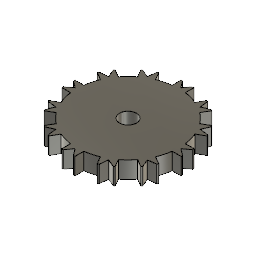
turn wheel v2 (Autodesk Fusion 360 design; units mm, degrees)
Autodesk Fusion 360 part; units mm, degrees
sketch "turn wheel" plane through (0, 0, 0) normal (0, 0, 1) x (1, 0, 0)
  circle A0 centre (0, 0) radius 30
  line L0 (-3.8635, 29.7502) -> (-3.8635, 35)
  line L1 (-3.8635, 35) -> (-3, 35)
  line L2 (-3, 35) -> (0, 31)
  line L3 (0, 35) -> (0, 30) construction
  line L4 (3.8635, 29.7502) -> (3.8635, 35)
  line L5 (3.8635, 35) -> (3, 35)
  line L6 (3, 35) -> (0, 31)
  line L7 (-18.2209, 23.8327) -> (-20.8458, 28.3792)
  line L8 (-20.0981, 28.8109) -> (-15.5, 26.8468)
  line L9 (-20.8458, 28.3792) -> (-20.0981, 28.8109)
  line L10 (-14.9019, 31.8109) -> (-15.5, 26.8468)
  line L11 (-14.1542, 32.2426) -> (-14.9019, 31.8109)
  line L12 (-11.5292, 27.6961) -> (-14.1542, 32.2426)
  line L13 (-27.6961, 11.5292) -> (-32.2426, 14.1542)
  line L14 (-31.8109, 14.9019) -> (-26.8468, 15.5)
  line L15 (-32.2426, 14.1542) -> (-31.8109, 14.9019)
  line L16 (-28.8109, 20.0981) -> (-26.8468, 15.5)
  line L17 (-28.3792, 20.8458) -> (-28.8109, 20.0981)
  line L18 (-23.8327, 18.2209) -> (-28.3792, 20.8458)
  line L19 (-29.7502, -3.8635) -> (-35, -3.8635)
  line L20 (-35, -3) -> (-31, 0)
  line L21 (-35, -3.8635) -> (-35, -3)
  line L22 (-35, 3) -> (-31, 0)
  line L23 (-35, 3.8635) -> (-35, 3)
  line L24 (-29.7502, 3.8635) -> (-35, 3.8635)
  line L25 (-23.8327, -18.2209) -> (-28.3792, -20.8458)
  line L26 (-28.8109, -20.0981) -> (-26.8468, -15.5)
  line L27 (-28.3792, -20.8458) -> (-28.8109, -20.0981)
  line L28 (-31.8109, -14.9019) -> (-26.8468, -15.5)
  line L29 (-32.2426, -14.1542) -> (-31.8109, -14.9019)
  line L30 (-27.6961, -11.5292) -> (-32.2426, -14.1542)
  line L31 (-11.5292, -27.6961) -> (-14.1542, -32.2426)
  line L32 (-14.9019, -31.8109) -> (-15.5, -26.8468)
  line L33 (-14.1542, -32.2426) -> (-14.9019, -31.8109)
  line L34 (-20.0981, -28.8109) -> (-15.5, -26.8468)
  line L35 (-20.8458, -28.3792) -> (-20.0981, -28.8109)
  line L36 (-18.2209, -23.8327) -> (-20.8458, -28.3792)
  line L37 (3.8635, -29.7502) -> (3.8635, -35)
  line L38 (3, -35) -> (0, -31)
  line L39 (3.8635, -35) -> (3, -35)
  line L40 (-3, -35) -> (0, -31)
  line L41 (-3.8635, -35) -> (-3, -35)
  line L42 (-3.8635, -29.7502) -> (-3.8635, -35)
  line L43 (18.2209, -23.8327) -> (20.8458, -28.3792)
  line L44 (20.0981, -28.8109) -> (15.5, -26.8468)
  line L45 (20.8458, -28.3792) -> (20.0981, -28.8109)
  line L46 (14.9019, -31.8109) -> (15.5, -26.8468)
  line L47 (14.1542, -32.2426) -> (14.9019, -31.8109)
  line L48 (11.5292, -27.6961) -> (14.1542, -32.2426)
  line L49 (27.6961, -11.5292) -> (32.2426, -14.1542)
  line L50 (31.8109, -14.9019) -> (26.8468, -15.5)
  line L51 (32.2426, -14.1542) -> (31.8109, -14.9019)
  line L52 (28.8109, -20.0981) -> (26.8468, -15.5)
  line L53 (28.3792, -20.8458) -> (28.8109, -20.0981)
  line L54 (23.8327, -18.2209) -> (28.3792, -20.8458)
  line L55 (29.7502, 3.8635) -> (35, 3.8635)
  line L56 (35, 3) -> (31, 0)
  line L57 (35, 3.8635) -> (35, 3)
  line L58 (35, -3) -> (31, 0)
  line L59 (35, -3.8635) -> (35, -3)
  line L60 (29.7502, -3.8635) -> (35, -3.8635)
  line L61 (23.8327, 18.2209) -> (28.3792, 20.8458)
  line L62 (28.8109, 20.0981) -> (26.8468, 15.5)
  line L63 (28.3792, 20.8458) -> (28.8109, 20.0981)
  line L64 (31.8109, 14.9019) -> (26.8468, 15.5)
  line L65 (32.2426, 14.1542) -> (31.8109, 14.9019)
  line L66 (27.6961, 11.5292) -> (32.2426, 14.1542)
  line L67 (11.5292, 27.6961) -> (14.1542, 32.2426)
  line L68 (14.9019, 31.8109) -> (15.5, 26.8468)
  line L69 (14.1542, 32.2426) -> (14.9019, 31.8109)
  line L70 (20.0981, 28.8109) -> (15.5, 26.8468)
  line L71 (20.8458, 28.3792) -> (20.0981, 28.8109)
  line L72 (18.2209, 23.8327) -> (20.8458, 28.3792)
  dimension "d1" = 60
  dimension "d2" = 5.2498
  dimension "d3" = 0.8635
  dimension "d4" = 5
  dimension "d6" = 360
  constraint coincident A0.centre origin
  constraint coincident A0 L0.start
  constraint vertical L0
  constraint perpendicular L0 L1
  constraint coincident A0 L3.end
  constraint vertical L3
  constraint symmetric L0.start L3 L4.start
  constraint symmetric L0.end L3 L4.end
  constraint symmetric L1.end L3 L5.end
  constraint symmetric L2.end L3 L6.end
  constraint perpendicular L4 L5
  measures "d1" diameter of A0
  measures "d2" distance of L0.start L0.end
  measures "d3" distance of L0.end L1.end
  measures "d4" distance of L1.end L2.end
extrude "Extrude1" add sketch "turn wheel" along normal blind 10
sketch "hole punch" plane through (0, 0, 10) normal (0, 0, 1) x (-1, 0, 0)
  arc A0 (-23.8327, -18.2209) -> (-18.2209, -23.8327) centre (0, 0) ccw
  line L0 (-18.2209, -23.8327) -> (-20.8458, -28.3792)
  line L1 (-20.8458, -28.3792) -> (-20.0981, -28.8109)
  line L2 (-20.0981, -28.8109) -> (-15.5, -26.8468)
  line L3 (-15.5, -26.8468) -> (-14.9019, -31.8109)
  line L4 (-14.9019, -31.8109) -> (-14.1542, -32.2426)
  line L5 (-14.1542, -32.2426) -> (-11.5292, -27.6961)
  arc A1 (-11.5292, -27.6961) -> (-3.8635, -29.7502) centre (0, 0) ccw
  line L6 (-3.8635, -29.7502) -> (-3.8635, -35)
  line L7 (-3.8635, -35) -> (-3, -35)
  line L8 (-3, -35) -> (0, -31)
  line L9 (0, -31) -> (3, -35)
  line L10 (3, -35) -> (3.8635, -35)
  line L11 (3.8635, -35) -> (3.8635, -29.7502)
  arc A2 (3.8635, -29.7502) -> (11.5292, -27.6961) centre (0, 0) ccw
  line L12 (11.5292, -27.6961) -> (14.1542, -32.2426)
  line L13 (14.1542, -32.2426) -> (14.9019, -31.8109)
  line L14 (14.9019, -31.8109) -> (15.5, -26.8468)
  line L15 (15.5, -26.8468) -> (20.0981, -28.8109)
  line L16 (20.0981, -28.8109) -> (20.8458, -28.3792)
  line L17 (20.8458, -28.3792) -> (18.2209, -23.8327)
  arc A3 (18.2209, -23.8327) -> (23.8327, -18.2209) centre (0, 0) ccw
  line L18 (23.8327, -18.2209) -> (28.3792, -20.8458)
  line L19 (28.3792, -20.8458) -> (28.8109, -20.0981)
  line L20 (28.8109, -20.0981) -> (26.8468, -15.5)
  line L21 (26.8468, -15.5) -> (31.8109, -14.9019)
  line L22 (31.8109, -14.9019) -> (32.2426, -14.1542)
  line L23 (32.2426, -14.1542) -> (27.6961, -11.5292)
  arc A4 (27.6961, -11.5292) -> (29.7502, -3.8635) centre (0, 0) ccw
  line L24 (29.7502, -3.8635) -> (35, -3.8635)
  line L25 (35, -3.8635) -> (35, -3)
  line L26 (35, -3) -> (31, 0)
  line L27 (31, 0) -> (35, 3)
  line L28 (35, 3) -> (35, 3.8635)
  line L29 (35, 3.8635) -> (29.7502, 3.8635)
  arc A5 (29.7502, 3.8635) -> (27.6961, 11.5292) centre (0, 0) ccw
  line L30 (27.6961, 11.5292) -> (32.2426, 14.1542)
  line L31 (32.2426, 14.1542) -> (31.8109, 14.9019)
  line L32 (31.8109, 14.9019) -> (26.8468, 15.5)
  line L33 (26.8468, 15.5) -> (28.8109, 20.0981)
  line L34 (28.8109, 20.0981) -> (28.3792, 20.8458)
  line L35 (28.3792, 20.8458) -> (23.8327, 18.2209)
  arc A6 (23.8327, 18.2209) -> (18.2209, 23.8327) centre (0, 0) ccw
  line L36 (18.2209, 23.8327) -> (20.8458, 28.3792)
  line L37 (20.8458, 28.3792) -> (20.0981, 28.8109)
  line L38 (20.0981, 28.8109) -> (15.5, 26.8468)
  line L39 (15.5, 26.8468) -> (14.9019, 31.8109)
  line L40 (14.9019, 31.8109) -> (14.1542, 32.2426)
  line L41 (14.1542, 32.2426) -> (11.5292, 27.6961)
  arc A7 (11.5292, 27.6961) -> (3.8635, 29.7502) centre (0, 0) ccw
  line L42 (3.8635, 29.7502) -> (3.8635, 35)
  line L43 (3.8635, 35) -> (3, 35)
  line L44 (3, 35) -> (0, 31)
  line L45 (0, 31) -> (-3, 35)
  line L46 (-3, 35) -> (-3.8635, 35)
  line L47 (-3.8635, 35) -> (-3.8635, 29.7502)
  arc A8 (-3.8635, 29.7502) -> (-11.5292, 27.6961) centre (0, 0) ccw
  line L48 (-11.5292, 27.6961) -> (-14.1542, 32.2426)
  line L49 (-14.1542, 32.2426) -> (-14.9019, 31.8109)
  line L50 (-14.9019, 31.8109) -> (-15.5, 26.8468)
  line L51 (-15.5, 26.8468) -> (-20.0981, 28.8109)
  line L52 (-20.0981, 28.8109) -> (-20.8458, 28.3792)
  line L53 (-20.8458, 28.3792) -> (-18.2209, 23.8327)
  arc A9 (-18.2209, 23.8327) -> (-23.8327, 18.2209) centre (0, 0) ccw
  line L54 (-23.8327, 18.2209) -> (-28.3792, 20.8458)
  line L55 (-28.3792, 20.8458) -> (-28.8109, 20.0981)
  line L56 (-28.8109, 20.0981) -> (-26.8468, 15.5)
  line L57 (-26.8468, 15.5) -> (-31.8109, 14.9019)
  line L58 (-31.8109, 14.9019) -> (-32.2426, 14.1542)
  line L59 (-32.2426, 14.1542) -> (-27.6961, 11.5292)
  arc A10 (-27.6961, 11.5292) -> (-29.7502, 3.8635) centre (0, 0) ccw
  line L60 (-29.7502, 3.8635) -> (-35, 3.8635)
  line L61 (-35, 3.8635) -> (-35, 3)
  line L62 (-35, 3) -> (-31, 0)
  line L63 (-31, 0) -> (-35, -3)
  line L64 (-35, -3) -> (-35, -3.8635)
  line L65 (-35, -3.8635) -> (-29.7502, -3.8635)
  arc A11 (-29.7502, -3.8635) -> (-27.6961, -11.5292) centre (0, 0) ccw
  line L66 (-27.6961, -11.5292) -> (-32.2426, -14.1542)
  line L67 (-32.2426, -14.1542) -> (-31.8109, -14.9019)
  line L68 (-31.8109, -14.9019) -> (-26.8468, -15.5)
  line L69 (-26.8468, -15.5) -> (-28.8109, -20.0981)
  line L70 (-28.8109, -20.0981) -> (-28.3792, -20.8458)
  line L71 (-28.3792, -20.8458) -> (-23.8327, -18.2209)
  line L72 (31, 0) -> (-31, 0) construction
  line L73 (0, -31) -> (0, 31) construction
  circle A12 centre (0, 0) radius 5
  constraint coincident L26.end L27.start
  constraint coincident L62.end L63.start
  constraint coincident L8.end L9.start
  constraint coincident L44.end L45.start
  constraint coincident A0.centre A1.centre
extrude "Extrude2" cut sketch "hole punch" against normal blind 10 contours A12
named bodies: "turn wheel"
